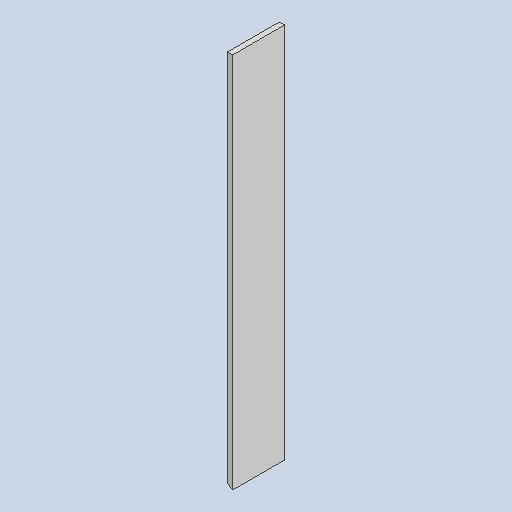
# Autodesk Inventor part: ДМФ 01 53 Боковая часть
Saved by Autodesk Inventor 2024.2 (Build 282272000, 272)
## iProperties
Created: 2024-05-05
Part Number: ДМФ 01 53 Боковая часть
Material: Generic
Document SubType Name: Modeling
Designer: pokla
Density: 1 g/cm^3
Appearance: Default
Author: pokla
Autodesk Inventor part; units mm, degrees
ref_plane "YZ Plane" through (0, 0, 0) normal (1, 0, 0) x (0, 1, 0)
ref_plane "XZ Plane" through (0, 0, 0) normal (0, 1, 0) x (-1, 0, 0)
ref_plane "XY Plane" through (0, 0, 0) normal (0, 0, 1) x (1, 0, 0)
sketch "Sketch1" plane through (0, 0, 0) normal (0, 0, 1) x (1, 0, 0)
  line L0 (0, 277.6336) -> (196.3166, 196.3166) construction
  line L1 (196.3166, 196.3166) -> (277.6336, 0) construction
  line L2 (277.6336, 0) -> (196.3166, -196.3166) construction
  line L3 (196.3166, -196.3166) -> (0, -277.6336) construction
  line L4 (0, -277.6336) -> (-196.3166, -196.3166) construction
  line L5 (-196.3166, -196.3166) -> (-277.6336, 0) construction
  line L6 (-277.6336, 0) -> (-196.3166, 196.3166) construction
  line L7 (-196.3166, 196.3166) -> (0, 277.6336) construction
  line L8 (-196.3166, 196.3166) -> (0, 277.6336) construction
  line L9 (-461.2666, 773.8898) -> (-221.0579, 873.3874) construction
  line L10 (-98.1583, 236.9751) -> (-341.1623, 823.6386) construction
  line L11 (-221.0579, 873.3874) -> (0, 873.3874) construction
  line L12 (0, 873.3874) -> (0, 277.6336) construction
  line L13 (-461.2666, 773.8898) -> (-617.5782, 617.5782) construction
  line L14 (-617.5782, 617.5782) -> (-196.3166, 196.3166) construction
  line L15 (-5, 280.9745) -> (-195.1434, 202.2145) construction
  line L16 (-195.1434, 202.2145) -> (-610.5071, 617.5782) construction
  line L17 (-610.5071, 617.5782) -> (-458.4343, 769.651) construction
  line L18 (-458.4343, 769.651) -> (-220.0634, 868.3874) construction
  line L19 (-220.0634, 868.3874) -> (-5, 868.3874) construction
  line L20 (-5, 868.3874) -> (-5, 280.9745) construction
  line L21 (-13, 286.3199) -> (-193.2664, 211.6511) construction
  line L22 (-193.2664, 211.6511) -> (-599.1934, 617.5782) construction
  line L23 (-599.1934, 617.5782) -> (-453.9027, 762.8689) construction
  line L24 (-453.9027, 762.8689) -> (-218.4721, 860.3874) construction
  line L25 (-218.4721, 860.3874) -> (-13, 860.3874) construction
  line L26 (-13, 860.3874) -> (-13, 286.3199) construction
  line L27 (-13, 860.3874) -> (-5, 860.3874)
  line L28 (-5, 860.3874) -> (-5, 280.9745)
  line L29 (-5, 280.9745) -> (-13, 286.3199)
  line L30 (-13, 286.3199) -> (-13, 860.3874)
  point P0 (0, 0)
  point P1 (0, 0)
  point P2 (0, 0)
  dimension "d0" = 513
  dimension "d1" = 260
  dimension "d2" = 635
  dimension "d10" = 5
  dimension "d11" = 8
  constraints: 62 end point, 3 perpendicular, 2 coincident, 2 midpoint, 1 collinear, 1 horizontal, 1 parallel, 1 point on line, 1 symmetric about line, 1 vertical, 1 vertical alignment, 27 other
  measures "d0" distance between parallel lines of L5 L1
  measures "d1" distance of L13.start L11.start
  measures "d2" distance of L10.end L10.start
  measures "d10" distance between parallel lines of L12 L20
  measures "d11" distance between parallel lines of L20 L26
extrude "Extrusion1" add sketch "Sketch1" against normal blind 80
equation "\"d0\" = Барабан_габарит_по_кассетам"
equation "\"d1\" = Кассета_длина_грани"
equation "\"d2\" = Кассета_высота"
equation "\"Барабан_габарит_по_кассетам\" = 513"
equation "\"Кассета_длина_грани\" = 260"
equation "\"Кассета_высота\" = 635"
body "Solid1"
